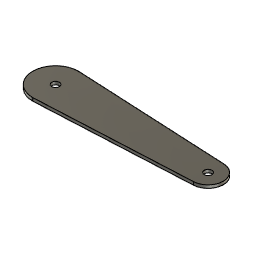
ANTEBRAZO v4 (Autodesk Fusion 360 design; units mm, degrees)
Autodesk Fusion 360 part; units mm, degrees
sketch "Boceto1" plane through (0, 0, 0) normal (0, 0, 1) x (1, 0, 0)
  circle A0 centre (0, 0) radius 30
  circle A1 centre (200, 0) radius 20
  line L0 (-0.0033, 30) -> (200.9963, 19.9752)
  line L1 (200.9963, -19.9752) -> (-0.0033, -30)
  circle A2 centre (0, 0) radius 5
  circle A3 centre (200, 0) radius 5
  constraint coincident A0.centre A2.centre
  constraint coincident A0 L0.start
  constraint coincident A1 L0.end
  constraint tangent A1 L0
  constraint coincident A1 L1.start
  constraint coincident A0 L1.end
  constraint tangent A1 L1
  constraint concentric A0 A2
  constraint concentric A1 A3
extrude "Extruir1" add sketch "Boceto1" along normal blind 4 contours A0 L0 L1 | A0 A1 L0 L1 | A1
sketch "Boceto2" plane through (0, 0, 4) normal (0, 0, 1) x (-1, 0, 0)
  circle A0 centre (-200, 0) radius 5
  circle A1 centre (0, 0) radius 5
  arc A2 (0.0033, -30) -> (0.0033, 30) centre (0, 0) ccw
  line L0 (0.0033, 30) -> (-200.9963, 19.9752)
  arc A3 (-200.9963, 19.9752) -> (-200.9963, -19.9752) centre (-200, 0) ccw
  line L1 (-200.9963, -19.9752) -> (0.0033, -30)
  line L2 (0, 0) -> (-40, 0)
  line L3 (-40, 0) -> (-80, 0)
  line L4 (-80, 0) -> (-120, 0)
  line L5 (-120, 0) -> (-160, 0)
  line L6 (-160, 0) -> (-200, 0)
  line L7 (0, 0) -> (15, 0)
  constraint coincident A1.centre A2.centre
  constraint horizontal L2
  constraint parallel L2 L3
  constraint parallel L3 L4
  constraint parallel L2 L7
